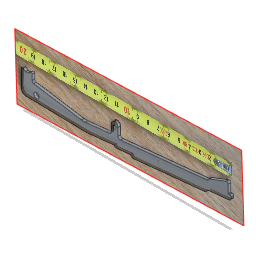
Trigger (Autodesk Fusion 360 design; units mm, degrees)
Autodesk Fusion 360 part; units mm, degrees
sketch "Sketch1" plane through (0, 0, 0) normal (0, 0, 1) x (1, 0, 0)
  line L0 (-66.4584, 0) -> (-66.4584, -10.2542)
  line L1 (-63.0659, -13.8981) -> (-24.9939, -14.6975)
  line L2 (-24.9939, -14.6975) -> (-7.7882, -12.8815)
  line L3 (-6.1483, -13.8071) -> (2.5452, -12.9249)
  line L4 (4.3444, -14.1925) -> (49.2418, -9.6793)
  line L5 (50.6036, -8.0187) -> (64.474, -6.6244)
  line L6 (63.9098, 1.6978) -> (63.9098, -3.4277)
  line L7 (63.9098, -3.4277) -> (64.771, -3.4277)
  line L8 (65.7451, -4.3959) -> (65.7451, -5.4039)
  spline S0 degree 5 poles (49.2418, -9.6793) (49.296, -9.6725) (49.402, -9.6567) (49.554, -9.6259) (49.7422, -9.5708) (49.9517, -9.4766) (50.1333, -9.3551) (50.2847, -9.204) (50.4049, -9.0222) (50.4952, -8.8112) (50.558, -8.5732) (50.588, -8.3629) (50.5999, -8.1948) (50.6032, -8.0781) (50.6036, -8.0187) knots 0 0 0 0 0 0 0.1 0.2 0.3 0.4 0.5 0.6 0.7 0.8 0.9 1 1 1 1 1 1
  spline S1 degree 5 poles (64.474, -6.6244) (64.515, -6.6203) (64.5956, -6.6103) (64.7125, -6.5901) (64.8601, -6.5522) (65.0296, -6.4854) (65.183, -6.3976) (65.3189, -6.2871) (65.4368, -6.153) (65.5374, -5.9964) (65.622, -5.819) (65.6781, -5.6618) (65.7139, -5.5359) (65.7351, -5.4485) (65.7451, -5.4039) knots 0 0 0 0 0 0 0.1 0.2 0.3 0.4 0.5 0.6 0.7 0.8 0.9 1 1 1 1 1 1
  spline S2 degree 5 poles (64.771, -3.4277) (64.8089, -3.4278) (64.8831, -3.4299) (64.9896, -3.438) (65.1217, -3.4591) (65.2694, -3.5036) (65.3981, -3.5679) (65.5062, -3.6536) (65.5928, -3.7616) (65.6589, -3.891) (65.706, -4.0402) (65.7298, -4.174) (65.7402, -4.282) (65.744, -4.3574) (65.7451, -4.3959) knots 0 0 0 0 0 0 0.1 0.2 0.3 0.4 0.5 0.6 0.7 0.8 0.9 1 1 1 1 1 1
  line L9 (51.7763, -1.4138) -> (62.5821, 2.6263)
  spline S3 degree 5 poles (62.5821, 2.6263) (62.6337, 2.643) (62.7346, 2.6732) (62.8794, 2.7094) (63.0592, 2.7388) (63.2602, 2.7422) (63.4355, 2.7092) (63.5828, 2.6369) (63.7011, 2.5236) (63.7914, 2.371) (63.8559, 2.1819) (63.8885, 2.0038) (63.903, 1.8562) (63.9083, 1.7517) (63.9098, 1.6978) knots 0 0 0 0 0 0 0.1 0.2 0.3 0.4 0.5 0.6 0.7 0.8 0.9 1 1 1 1 1 1
  line L10 (51.1753, -2.1665) -> (51.1753, -2.5504)
  line L11 (51.1753, -2.5504) -> (-3.7703, -8.0737)
  spline S4 degree 5 poles (51.1753, -2.1665) (51.1778, -2.1442) (51.1838, -2.1001) (51.1952, -2.036) (51.2155, -1.9544) (51.2498, -1.8593) (51.2939, -1.7717) (51.3485, -1.6922) (51.4141, -1.6212) (51.4903, -1.5583) (51.5762, -1.5029) (51.6521, -1.464) (51.7128, -1.4378) (51.7549, -1.4216) (51.7763, -1.4138) knots 0 0 0 0 0 0 0.1 0.2 0.3 0.4 0.5 0.6 0.7 0.8 0.9 1 1 1 1 1 1
  line L12 (-5.5189, -2.0779) -> (-5.5101, -6.9266)
  line L13 (-9.6729, -1.9196) -> (-9.7353, -6.8884)
  spline S5 degree 5 poles (-9.6729, -1.9196) (-9.6686, -1.8398) (-9.6571, -1.6837) (-9.6312, -1.4594) (-9.5793, -1.1807) (-9.4834, -0.8683) (-9.3537, -0.5952) (-9.1872, -0.3649) (-8.9821, -0.1795) (-8.7396, -0.0375) (-8.4624, 0.0641) (-8.2151, 0.1158) (-8.0162, 0.1389) (-7.8777, 0.1474) (-7.807, 0.15) knots 0 0 0 0 0 0 0.1 0.2 0.3 0.4 0.5 0.6 0.7 0.8 0.9 1 1 1 1 1 1
  spline S6 degree 5 poles (-5.5189, -2.0779) (-5.5279, -1.9856) (-5.5491, -1.8052) (-5.5905, -1.547) (-5.665, -1.2279) (-5.7927, -0.8739) (-5.9581, -0.5689) (-6.1645, -0.3171) (-6.414, -0.1211) (-6.7051, 0.0209) (-7.0349, 0.1126) (-7.3271, 0.1491) (-7.5613, 0.157) (-7.724, 0.1537) (-7.807, 0.15) knots 0 0 0 0 0 0 0.1 0.2 0.3 0.4 0.5 0.6 0.7 0.8 0.9 1 1 1 1 1 1
  spline S7 degree 5 poles (-5.5101, -6.9266) (-5.5029, -6.985) (-5.4862, -7.0986) (-5.4538, -7.2597) (-5.3959, -7.4555) (-5.2971, -7.6666) (-5.1697, -7.8409) (-5.0113, -7.9756) (-4.821, -8.0694) (-4.6, -8.1238) (-4.3507, -8.1421) (-4.1306, -8.1302) (-3.9546, -8.1073) (-3.8325, -8.0859) (-3.7703, -8.0737) knots 0 0 0 0 0 0 0.1 0.2 0.3 0.4 0.5 0.6 0.7 0.8 0.9 1 1 1 1 1 1
  spline S8 degree 5 poles (-7.7882, -12.8815) (-7.7811, -12.9256) (-7.7646, -13.0114) (-7.7329, -13.1335) (-7.6768, -13.2823) (-7.582, -13.4438) (-7.4605, -13.5787) (-7.3102, -13.6849) (-7.1304, -13.7618) (-6.9227, -13.8108) (-6.6893, -13.8342) (-6.4838, -13.8342) (-6.3198, -13.8244) (-6.2062, -13.8136) (-6.1483, -13.8071) knots 0 0 0 0 0 0 0.1 0.2 0.3 0.4 0.5 0.6 0.7 0.8 0.9 1 1 1 1 1 1
  spline S9 degree 5 poles (2.5452, -12.9249) (2.5562, -12.9845) (2.5804, -13.1007) (2.6233, -13.2661) (2.6937, -13.4684) (2.8055, -13.6887) (2.9431, -13.8736) (3.1086, -14.0201) (3.3031, -14.1269) (3.5254, -14.1955) (3.7735, -14.2287) (3.9909, -14.2293) (4.1638, -14.2162) (4.2835, -14.2014) (4.3444, -14.1925) knots 0 0 0 0 0 0 0.1 0.2 0.3 0.4 0.5 0.6 0.7 0.8 0.9 1 1 1 1 1 1
  line L14 (-10.8955, -7.8607) -> (-26.0915, -9.4536)
  spline S10 degree 5 poles (-9.7353, -6.8884) (-9.7444, -6.9253) (-9.7639, -6.9976) (-9.7969, -7.1015) (-9.8483, -7.2307) (-9.9259, -7.3757) (-10.018, -7.5026) (-10.1258, -7.6101) (-10.25, -7.6972) (-10.3899, -7.7648) (-10.5443, -7.8143) (-10.6786, -7.8406) (-10.7849, -7.8533) (-10.8582, -7.8588) (-10.8955, -7.8607) knots 0 0 0 0 0 0 0.1 0.2 0.3 0.4 0.5 0.6 0.7 0.8 0.9 1 1 1 1 1 1
  line L15 (-58.618, -4.675) -> (-28.5127, -9.4217)
  spline S11 degree 5 poles (-28.5127, -9.4217) (-28.4572, -9.4307) (-28.3469, -9.448) (-28.1832, -9.4717) (-27.9686, -9.499) (-27.707, -9.5252) (-27.4526, -9.5429) (-27.2061, -9.5512) (-26.9679, -9.5498) (-26.7377, -9.5389) (-26.5151, -9.5191) (-26.3424, -9.4967) (-26.2159, -9.4765) (-26.1328, -9.4615) (-26.0915, -9.4536) knots 0 0 0 0 0 0 0.1 0.2 0.3 0.4 0.5 0.6 0.7 0.8 0.9 1 1 1 1 1 1
  line L16 (-59.51, -3.5281) -> (-59.51, 0)
  spline S12 degree 5 poles (-59.51, -3.5281) (-59.51, -3.5685) (-59.5086, -3.6476) (-59.5017, -3.7618) (-59.483, -3.9049) (-59.4429, -4.0673) (-59.3843, -4.2118) (-59.3057, -4.3368) (-59.2063, -4.4416) (-59.0868, -4.5268) (-58.9486, -4.5938) (-58.8244, -4.634) (-58.7239, -4.6572) (-58.6538, -4.6696) (-58.618, -4.675) knots 0 0 0 0 0 0 0.1 0.2 0.3 0.4 0.5 0.6 0.7 0.8 0.9 1 1 1 1 1 1
  spline S13 degree 5 poles (-66.4584, -10.2542) (-66.4543, -10.3931) (-66.4406, -10.6651) (-66.4035, -11.056) (-66.3201, -11.5421) (-66.1557, -12.0875) (-65.9256, -12.5649) (-65.6244, -12.9686) (-65.2488, -13.2954) (-64.8014, -13.5478) (-64.2874, -13.7313) (-63.8273, -13.8275) (-63.4564, -13.873) (-63.1979, -13.8917) (-63.0659, -13.8981) knots 0 0 0 0 0 0 0.1 0.2 0.3 0.4 0.5 0.6 0.7 0.8 0.9 1 1 1 1 1 1
  line L17 (-65.2339, 0.2746) -> (-63.5697, -0.646)
  line L18 (-62.2949, -0.646) -> (-60.8077, 0.2038)
  spline S14 degree 5 poles (-63.5697, -0.646) (-63.5442, -0.6632) (-63.4934, -0.6959) (-63.417, -0.7405) (-63.3152, -0.7909) (-63.1879, -0.8377) (-63.0606, -0.8667) (-62.9331, -0.8767) (-62.8056, -0.8667) (-62.678, -0.8376) (-62.5504, -0.7909) (-62.4482, -0.7405) (-62.3716, -0.6959) (-62.3205, -0.6631) (-62.2949, -0.646) knots 0 0 0 0 0 0 0.1 0.2 0.3 0.4 0.5 0.6 0.7 0.8 0.9 1 1 1 1 1 1
  spline S15 degree 5 poles (-66.4584, 0) (-66.452, 0.0346) (-66.4375, 0.1013) (-66.4109, 0.1935) (-66.3657, 0.3007) (-66.2918, 0.4066) (-66.1991, 0.4821) (-66.0862, 0.5249) (-65.9526, 0.5343) (-65.7994, 0.5121) (-65.6282, 0.4609) (-65.4781, 0.3987) (-65.3587, 0.3409) (-65.276, 0.2975) (-65.2339, 0.2746) knots 0 0 0 0 0 0 0.1 0.2 0.3 0.4 0.5 0.6 0.7 0.8 0.9 1 1 1 1 1 1
  spline S16 degree 5 poles (-60.8077, 0.2038) (-60.7594, 0.2307) (-60.6646, 0.2818) (-60.5282, 0.3506) (-60.3578, 0.4263) (-60.1656, 0.4922) (-59.9962, 0.5267) (-59.8516, 0.5269) (-59.7334, 0.4904) (-59.6414, 0.4178) (-59.5737, 0.3115) (-59.5377, 0.2015) (-59.5202, 0.1058) (-59.5127, 0.0362) (-59.51, 0) knots 0 0 0 0 0 0 0.1 0.2 0.3 0.4 0.5 0.6 0.7 0.8 0.9 1 1 1 1 1 1
  point P0 (50.2693, -9.2056)
  point P1 (65.3076, -6.2877)
  point P2 (65.5, -3.6584)
  point P3 (63.5761, 2.6263)
  point P4 (51.351, -1.6947)
  point P5 (-9.1597, -0.3566)
  point P6 (-6.1971, -0.31)
  point P7 (-5.013, -7.959)
  point P8 (-7.3299, -13.662)
  point P9 (3.1139, -14.0089)
  point P10 (-10.1309, -7.6059)
  point P11 (-27.1747, -9.5492)
  point P12 (-59.2958, -4.3378)
  point P13 (-65.588, -12.9685)
  point P14 (-62.9333, -0.8717)
  point P15 (-66.1038, 0.5111)
  point P16 (-59.8219, 0.5111)
  constraint vertical L0
  constraint parallel L4 L5
  constraint vertical L6
  constraint perpendicular L6 L7
  constraint vertical L8
  constraint vertical L10
  constraint parallel L4 L11
  constraint vertical L16
extrude "Extrude1" add sketch "Sketch1" along normal blind 1.7
hole "Hole1" at (-7.5758, -2.9708, 1.7) direction (0, 0, -1) diameter 2 depth 15 tip angle 118
sketch "Sketch2" plane through (0, 0, 1.7) normal (0, 0, 1) x (1, 0, 0)
  circle A0 centre (-7.5758, -2.9708) radius 1
  line L0 (-66.4584, 0) -> (-66.4584, -10.2542)
  spline S0 degree 5 poles (-66.4584, -10.2542) (-66.4543, -10.3931) (-66.4406, -10.6651) (-66.4035, -11.056) (-66.3201, -11.5421) (-66.1557, -12.0875) (-65.9256, -12.5649) (-65.6244, -12.9686) (-65.2488, -13.2954) (-64.8014, -13.5478) (-64.2874, -13.7313) (-63.8273, -13.8275) (-63.4564, -13.873) (-63.1979, -13.8917) (-63.0659, -13.8981) knots 0 0 0 0 0 0 0.1 0.2 0.3 0.4 0.5 0.6 0.7 0.8 0.9 1 1 1 1 1 1
  line L1 (-63.0659, -13.8981) -> (-24.9939, -14.6975)
  line L2 (-24.9939, -14.6975) -> (-7.7882, -12.8815)
  spline S1 degree 5 poles (-7.7882, -12.8815) (-7.7811, -12.9256) (-7.7646, -13.0114) (-7.7329, -13.1335) (-7.6768, -13.2823) (-7.582, -13.4438) (-7.4605, -13.5787) (-7.3102, -13.6849) (-7.1304, -13.7618) (-6.9227, -13.8108) (-6.6893, -13.8342) (-6.4838, -13.8342) (-6.3198, -13.8244) (-6.2062, -13.8136) (-6.1483, -13.8071) knots 0 0 0 0 0 0 0.1 0.2 0.3 0.4 0.5 0.6 0.7 0.8 0.9 1 1 1 1 1 1
  line L3 (-6.1483, -13.8071) -> (2.5452, -12.9249)
  spline S2 degree 5 poles (2.5452, -12.9249) (2.5562, -12.9845) (2.5804, -13.1007) (2.6233, -13.2661) (2.6937, -13.4684) (2.8055, -13.6887) (2.9431, -13.8736) (3.1086, -14.0201) (3.3031, -14.1269) (3.5254, -14.1955) (3.7735, -14.2287) (3.9909, -14.2293) (4.1638, -14.2162) (4.2835, -14.2014) (4.3444, -14.1925) knots 0 0 0 0 0 0 0.1 0.2 0.3 0.4 0.5 0.6 0.7 0.8 0.9 1 1 1 1 1 1
  line L4 (4.3444, -14.1925) -> (49.2418, -9.6793)
  spline S3 degree 5 poles (49.2418, -9.6793) (49.296, -9.6725) (49.402, -9.6567) (49.554, -9.6259) (49.7422, -9.5708) (49.9517, -9.4766) (50.1333, -9.3551) (50.2847, -9.204) (50.4049, -9.0222) (50.4952, -8.8112) (50.558, -8.5732) (50.588, -8.3629) (50.5999, -8.1948) (50.6032, -8.0781) (50.6036, -8.0187) knots 0 0 0 0 0 0 0.1 0.2 0.3 0.4 0.5 0.6 0.7 0.8 0.9 1 1 1 1 1 1
  line L5 (50.6036, -8.0187) -> (64.474, -6.6244)
  spline S4 degree 5 poles (64.474, -6.6244) (64.515, -6.6203) (64.5956, -6.6103) (64.7125, -6.5901) (64.8601, -6.5522) (65.0296, -6.4854) (65.183, -6.3976) (65.3189, -6.2871) (65.4368, -6.153) (65.5374, -5.9964) (65.622, -5.819) (65.6781, -5.6618) (65.7139, -5.5359) (65.7351, -5.4485) (65.7451, -5.4039) knots 0 0 0 0 0 0 0.1 0.2 0.3 0.4 0.5 0.6 0.7 0.8 0.9 1 1 1 1 1 1
  line L6 (65.7451, -5.4039) -> (65.7451, -4.3959)
  spline S5 degree 5 poles (65.7451, -4.3959) (65.744, -4.3574) (65.7402, -4.282) (65.7298, -4.174) (65.706, -4.0402) (65.6589, -3.891) (65.5928, -3.7616) (65.5062, -3.6536) (65.3981, -3.5679) (65.2694, -3.5036) (65.1217, -3.4591) (64.9896, -3.438) (64.8831, -3.4299) (64.8089, -3.4278) (64.771, -3.4277) knots -1 -1 -1 -1 -1 -1 -0.9 -0.8 -0.7 -0.6 -0.5 -0.4 -0.3 -0.2 -0.1 0 0 0 0 0 0
  line L7 (64.771, -3.4277) -> (63.9098, -3.4277)
  line L8 (63.9098, -3.4277) -> (63.9098, 1.6978)
  spline S6 degree 5 poles (63.9098, 1.6978) (63.9083, 1.7517) (63.903, 1.8562) (63.8885, 2.0038) (63.8559, 2.1819) (63.7914, 2.371) (63.7011, 2.5236) (63.5828, 2.6369) (63.4355, 2.7092) (63.2602, 2.7422) (63.0592, 2.7388) (62.8794, 2.7094) (62.7346, 2.6732) (62.6337, 2.643) (62.5821, 2.6263) knots -1 -1 -1 -1 -1 -1 -0.9 -0.8 -0.7 -0.6 -0.5 -0.4 -0.3 -0.2 -0.1 0 0 0 0 0 0
  line L9 (62.5821, 2.6263) -> (51.7763, -1.4138)
  spline S7 degree 5 poles (51.7763, -1.4138) (51.7549, -1.4216) (51.7128, -1.4378) (51.6521, -1.464) (51.5762, -1.5029) (51.4903, -1.5583) (51.4141, -1.6212) (51.3485, -1.6922) (51.2939, -1.7717) (51.2498, -1.8593) (51.2155, -1.9544) (51.1952, -2.036) (51.1838, -2.1001) (51.1778, -2.1442) (51.1753, -2.1665) knots -1 -1 -1 -1 -1 -1 -0.9 -0.8 -0.7 -0.6 -0.5 -0.4 -0.3 -0.2 -0.1 0 0 0 0 0 0
  line L10 (51.1753, -2.1665) -> (51.1753, -2.5504)
  line L11 (51.1753, -2.5504) -> (-3.7703, -8.0737)
  spline S8 degree 5 poles (-3.7703, -8.0737) (-3.8325, -8.0859) (-3.9546, -8.1073) (-4.1306, -8.1302) (-4.3507, -8.1421) (-4.6, -8.1238) (-4.821, -8.0694) (-5.0113, -7.9756) (-5.1697, -7.8409) (-5.2971, -7.6666) (-5.3959, -7.4555) (-5.4538, -7.2597) (-5.4862, -7.0986) (-5.5029, -6.985) (-5.5101, -6.9266) knots -1 -1 -1 -1 -1 -1 -0.9 -0.8 -0.7 -0.6 -0.5 -0.4 -0.3 -0.2 -0.1 0 0 0 0 0 0
  line L12 (-5.5101, -6.9266) -> (-5.5189, -2.0779)
  spline S9 degree 5 poles (-5.5189, -2.0779) (-5.5279, -1.9856) (-5.5491, -1.8052) (-5.5905, -1.547) (-5.665, -1.2279) (-5.7927, -0.8739) (-5.9581, -0.5689) (-6.1645, -0.3171) (-6.414, -0.1211) (-6.7051, 0.0209) (-7.0349, 0.1126) (-7.3271, 0.1491) (-7.5613, 0.157) (-7.724, 0.1537) (-7.807, 0.15) knots 0 0 0 0 0 0 0.1 0.2 0.3 0.4 0.5 0.6 0.7 0.8 0.9 1 1 1 1 1 1
  spline S10 degree 5 poles (-7.807, 0.15) (-7.8777, 0.1474) (-8.0162, 0.1389) (-8.2151, 0.1158) (-8.4624, 0.0641) (-8.7396, -0.0375) (-8.9821, -0.1795) (-9.1872, -0.3649) (-9.3537, -0.5952) (-9.4834, -0.8683) (-9.5793, -1.1807) (-9.6312, -1.4594) (-9.6571, -1.6837) (-9.6686, -1.8398) (-9.6729, -1.9196) knots -1 -1 -1 -1 -1 -1 -0.9 -0.8 -0.7 -0.6 -0.5 -0.4 -0.3 -0.2 -0.1 0 0 0 0 0 0
  line L13 (-9.6729, -1.9196) -> (-9.7353, -6.8884)
  spline S11 degree 5 poles (-9.7353, -6.8884) (-9.7444, -6.9253) (-9.7639, -6.9976) (-9.7969, -7.1015) (-9.8483, -7.2307) (-9.9259, -7.3757) (-10.018, -7.5026) (-10.1258, -7.6101) (-10.25, -7.6972) (-10.3899, -7.7648) (-10.5443, -7.8143) (-10.6786, -7.8406) (-10.7849, -7.8533) (-10.8582, -7.8588) (-10.8955, -7.8607) knots 0 0 0 0 0 0 0.1 0.2 0.3 0.4 0.5 0.6 0.7 0.8 0.9 1 1 1 1 1 1
  line L14 (-10.8955, -7.8607) -> (-26.0915, -9.4536)
  spline S12 degree 5 poles (-26.0915, -9.4536) (-26.1328, -9.4615) (-26.2159, -9.4765) (-26.3424, -9.4967) (-26.5151, -9.5191) (-26.7377, -9.5389) (-26.9679, -9.5498) (-27.2061, -9.5512) (-27.4526, -9.5429) (-27.707, -9.5252) (-27.9686, -9.499) (-28.1832, -9.4717) (-28.3469, -9.448) (-28.4572, -9.4307) (-28.5127, -9.4217) knots -1 -1 -1 -1 -1 -1 -0.9 -0.8 -0.7 -0.6 -0.5 -0.4 -0.3 -0.2 -0.1 0 0 0 0 0 0
  line L15 (-28.5127, -9.4217) -> (-58.618, -4.675)
  spline S13 degree 5 poles (-58.618, -4.675) (-58.6538, -4.6696) (-58.7239, -4.6572) (-58.8244, -4.634) (-58.9486, -4.5938) (-59.0868, -4.5268) (-59.2063, -4.4416) (-59.3057, -4.3368) (-59.3843, -4.2118) (-59.4429, -4.0673) (-59.483, -3.9049) (-59.5017, -3.7618) (-59.5086, -3.6476) (-59.51, -3.5685) (-59.51, -3.5281) knots -1 -1 -1 -1 -1 -1 -0.9 -0.8 -0.7 -0.6 -0.5 -0.4 -0.3 -0.2 -0.1 0 0 0 0 0 0
  line L16 (-59.51, -3.5281) -> (-59.51, 0)
  spline S14 degree 5 poles (-59.51, 0) (-59.5127, 0.0362) (-59.5202, 0.1058) (-59.5377, 0.2015) (-59.5737, 0.3115) (-59.6414, 0.4178) (-59.7334, 0.4904) (-59.8516, 0.5269) (-59.9962, 0.5267) (-60.1656, 0.4922) (-60.3578, 0.4263) (-60.5282, 0.3506) (-60.6646, 0.2818) (-60.7594, 0.2307) (-60.8077, 0.2038) knots -1 -1 -1 -1 -1 -1 -0.9 -0.8 -0.7 -0.6 -0.5 -0.4 -0.3 -0.2 -0.1 0 0 0 0 0 0
  line L17 (-60.8077, 0.2038) -> (-62.2949, -0.646)
  spline S15 degree 5 poles (-62.2949, -0.646) (-62.3205, -0.6631) (-62.3716, -0.6959) (-62.4482, -0.7405) (-62.5504, -0.7909) (-62.678, -0.8376) (-62.8056, -0.8667) (-62.9331, -0.8767) (-63.0606, -0.8667) (-63.1879, -0.8377) (-63.3152, -0.7909) (-63.417, -0.7405) (-63.4934, -0.6959) (-63.5442, -0.6632) (-63.5697, -0.646) knots -1 -1 -1 -1 -1 -1 -0.9 -0.8 -0.7 -0.6 -0.5 -0.4 -0.3 -0.2 -0.1 0 0 0 0 0 0
  line L18 (-63.5697, -0.646) -> (-65.2339, 0.2746)
  spline S16 degree 5 poles (-65.2339, 0.2746) (-65.276, 0.2975) (-65.3587, 0.3409) (-65.4781, 0.3987) (-65.6282, 0.4609) (-65.7994, 0.5121) (-65.9526, 0.5343) (-66.0862, 0.5249) (-66.1991, 0.4821) (-66.2918, 0.4066) (-66.3657, 0.3007) (-66.4109, 0.1935) (-66.4375, 0.1013) (-66.452, 0.0346) (-66.4584, 0) knots -1 -1 -1 -1 -1 -1 -0.9 -0.8 -0.7 -0.6 -0.5 -0.4 -0.3 -0.2 -0.1 0 0 0 0 0 0
  circle A1 centre (-56.7832, -10.2874) radius 1.7
  dimension "d6" = 3.4
  measures "d6" diameter of A1
extrude "Extrude2" cut sketch "Sketch2" against normal blind 3 contours A1
